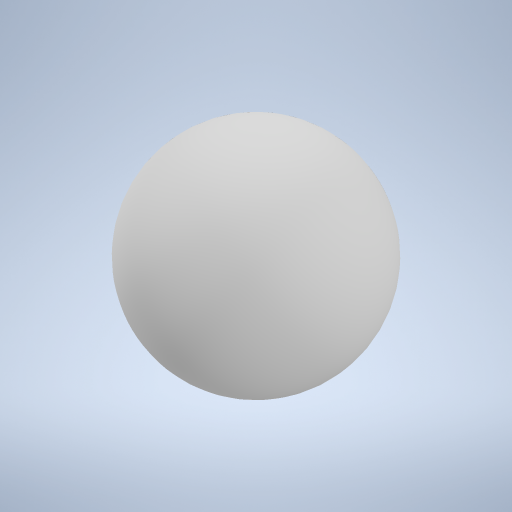
# Autodesk Inventor part: Hudson 1-58
Saved by Autodesk Inventor 2024.2 (Build 282272000, 272)
## iProperties
Created: 2024-10-06
Part Number: Hudson 1-58
Material: Genérico
Document SubType Name: Modeling
Designer: Monica Mora
Density: 1 g/cm^3
Appearance: Valor por defecto
Author: Monica Mora
Autodesk Inventor part; units mm, degrees
ref_plane "YZ Plane" through (0, 0, 0) normal (1, 0, 0) x (0, 1, 0)
ref_plane "XZ Plane" through (0, 0, 0) normal (0, 1, 0) x (-1, 0, 0)
ref_plane "XY Plane" through (0, 0, 0) normal (0, 0, 1) x (1, 0, 0)
sketch "Boceto1" plane through (0, 0, 0) normal (0, 0, 1) x (1, 0, 0)
  circle A0 centre (0, 0) radius 2.5
  circle A1 centre (0, 0) radius 2.25
  line L0 (2.9119, 0) -> (-3.7877, 0)
  point P0 (-2.5, 0)
  point P1 (2.5, 0)
  point P2 (-2.25, 0)
  point P3 (2.25, 0)
  dimension "d0" = 5
  dimension "d1" = 4.5
  constraints: 2 centre point, 2 coincident, 2 end point, 1 horizontal
  measures "d0" diameter of A0
  measures "d1" diameter of A1
revolve "Revolución1" add sketch "Boceto1" angle 360 about axis through (2.9119, 0, 0) along (-1, 0, 0) picked at (-2.3707, 0.3789) contours L0 A1 A0
